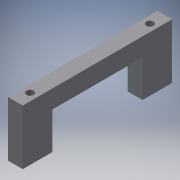
# Autodesk Inventor part: Intake Robustifier
Saved by Autodesk Inventor 2018 (Build 220112000, 112)
## iProperties
Created: 2018-02-10
Part Number: Intake Robustifier
Material: Generic
Document SubType Name: Modeling
Designer: Orangeracer
Density: 1 g/cm^3
Appearance: Default
Author: Orangeracer
Autodesk Inventor part; units mm, degrees
ref_plane "YZ Plane" through (0, 0, 0) normal (1, 0, 0) x (0, 1, 0)
ref_plane "XZ Plane" through (0, 0, 0) normal (0, 1, 0) x (-1, 0, 0)
ref_plane "XY Plane" through (0, 0, 0) normal (0, 0, 1) x (1, 0, 0)
sketch "Sketch1" plane through (0, 0, 0) normal (0, 0, 1) x (1, 0, 0)
  line L0 (0, 0) -> (-12.7, 0)
  line L1 (-12.7, 0) -> (-12.7, 47.4345)
  line L2 (-12.7, 47.4345) -> (0, 47.4345)
  line L3 (0, 47.4345) -> (0, 0)
  dimension "d0" = 12.7
  dimension "d1" = 47.4345
  constraints: 8 end point, 2 parallel, 1 horizontal, 1 perpendicular
  measures "d0" distance of L1.end L2.end
  measures "d1" distance of L0.end L1.end
extrude "Extrusion1" add sketch "Sketch1" along normal blind 128.5875
sketch "Sketch2" plane through (0, 0, 0) normal (1, 0, 0) x (0, 0, -1)
  line L0 (-25.4, 0) -> (-103.1875, 0)
  line L1 (-103.1875, 0) -> (-103.1875, 31.75)
  line L2 (-103.1875, 31.75) -> (-25.4, 31.75)
  line L3 (-25.4, 31.75) -> (-25.4, 0)
  line L4 (0, 47.4345) -> (0, 0) projected
  line L5 (-128.5875, 0) -> (-128.5875, 47.4345) projected
  line L6 (0, 0) -> (-128.5875, 0) projected
  dimension "d4" = 25.4
  dimension "d5" = 25.4
  dimension "d6" = 77.7875
  dimension "d7" = 31.75
  dimension "d8" = 0
  constraints: 8 end point, 2 parallel, 1 horizontal, 1 perpendicular
  measures "d4" distance between parallel lines of L4 L3
  measures "d5" distance between parallel lines of L5 L1
  measures "d6" distance between parallel lines of L1 L3
  measures "d7" distance between parallel lines of L2 L0
  measures "d8" distance between parallel lines of L6 L0
extrude "Extrusion2" cut sketch "Sketch2" against normal blind 77.7875
sketch "Sketch3" plane through (-12.7, 47.4345, 0) normal (0, 1, 0) x (1, 0, 0)
  circle A0 centre (6.35, -115.8875) radius 3.175
  circle A1 centre (6.35, -12.7) radius 3.175
  line L0 (0, 0) -> (0, -128.5875) projected
  line L1 (12.7, -128.5875) -> (0, -128.5875) projected
  line L2 (0, 0) -> (12.7, 0) projected
  dimension "d11" = 6.35
  dimension "d12" = 6.35
  dimension "d13" = 6.35
  dimension "d14" = 6.35
  dimension "d15" = 12.7
  dimension "d16" = 12.7
  constraints: 2 centre point
  measures "d11" diameter of A0
  measures "d12" diameter of A1
  measures "d13" distance from line of A1.centre L0
  measures "d14" distance from line of A0.centre L0
  measures "d15" distance from line of A0.centre L1
  measures "d16" distance from line of A1.centre L2
extrude "Extrusion3" cut sketch "Sketch3" against normal blind 77.7875
chamfer "Chamfer1" distance 19.05 angle 45 2 edges at (-6.35, 47.4345, 0) (-6.35, 47.4345, 128.5875)
body "Solid1"
